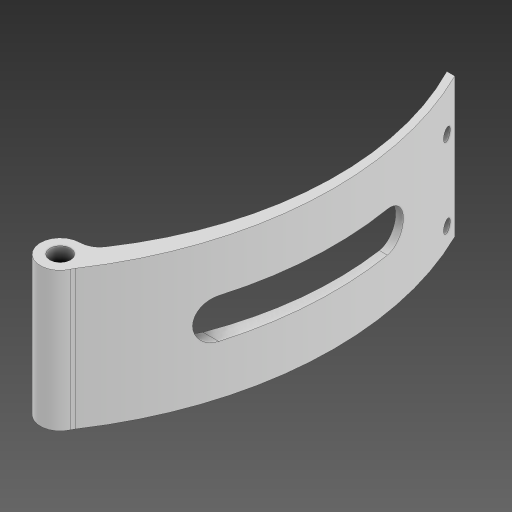
# Autodesk Inventor part: protect_2
Saved by Autodesk Inventor 2023 (Build 270158000, 158)
## iProperties
Created: 2025-06-27
Part Number: protect_2
Material: Типовые
Document SubType Name: Modeling
Designer: daa
Density: 1 g/cm^3
Appearance: По умолчанию
Author: daa
Autodesk Inventor part; units mm, degrees
ref_plane "YZ Plane" through (0, 0, 0) normal (1, 0, 0) x (0, 1, 0)
ref_plane "XZ Plane" through (0, 0, 0) normal (0, 1, 0) x (-1, 0, 0)
ref_plane "XY Plane" through (0, 0, 0) normal (0, 0, 1) x (1, 0, 0)
sketch "Эскиз1" plane through (0, 0, 0) normal (0, 1, 0) x (-1, 0, 0)
  circle A0 centre (-56.0718, 132.2835) radius 2.6
  line L0 (-64.9084, 43.85) -> (-66.9084, 43.85)
  circle A1 centre (-56.0718, 132.2835) radius 5.0026
  arc A2 (-60.8228, 133.85) -> (-66.9084, 43.85) centre (13.8399, 83.5958) ccw
  arc A3 (-58.2432, 127.7768) -> (-64.9084, 43.85) centre (6.2398, 80.4278) ccw
  line L1 (-60.8228, 133.85) -> (-51.3208, 133.85)
  point P0 (-68.2724, 116.2724)
  dimension "d27" = 5.2
  dimension "d28" = 2
  dimension "d29" = 90
  dimension "d30" = 80
  dimension "d35" = 90
  dimension "d47" = 10.0052
  dimension "d48" = 1.5665
  constraints: 7 point on circle, 4 centre point, 4 end point, 2 coincident, 2 horizontal
  measures "d27" diameter of A0
  measures "d28" distance of L0.start L0.end
  measures "d29" radius of A2
  measures "d30" radius of A3
  measures "d35" vertical distance of L0.end L1.start
  measures "d47" diameter of A1
  measures "d48" distance from line of L1 A0.centre
extrude "Выдавливание1" add sketch "Эскиз1" along normal blind 35 contours A0 L1 A1 | A0 L1 A1 | A1 A3 L0 A2
sketch "Эскиз2" plane through (0, 0, 0) normal (1, 0, 0) x (0, 1, 0)
  circle A0 centre (25, 47.55) radius 1.5
  circle A1 centre (5, 47.55) radius 1.5
  line L0 (0, 43.85) -> (35, 43.85) projected
  line L1 (35, 127.7768) -> (35, 43.85) projected
  line L2 (17.5, 68.85) -> (17.5, 108.85) construction
  line L3 (22.5, 68.85) -> (22.5, 108.85)
  line L4 (12.5, 108.85) -> (12.5, 68.85)
  arc A2 (12.5, 68.85) -> (22.5, 68.85) centre (17.5, 68.85) ccw
  arc A3 (22.5, 108.85) -> (12.5, 108.85) centre (17.5, 108.85) ccw
  point P0 (0, 0)
  point P1 (17.5, 88.85)
  point P2 (17.5, 63.85)
  dimension "d36" = 3
  dimension "d37" = 3
  dimension "d38" = 3.7
  dimension "d39" = 3.7
  dimension "d40" = 10
  dimension "d41" = 20
  dimension "d44" = 40
  dimension "d45" = 10
  dimension "d46" = 20
  constraints: 8 end point, 5 point on circle, 4 centre point, 4 tangent, 1 midpoint, 1 parallel, 1 vertical
  measures "d36" diameter of A0
  measures "d37" diameter of A1
  measures "d38" distance from line of L0 A1.centre
  measures "d39" distance from line of L0 A0.centre
  measures "d40" distance from line of L1 A0.centre
  measures "d41" distance of A0.centre A1.centre
  measures "d44" distance of L2.start L2.end
  measures "d45" diameter of A3
  measures "d46" distance from line of point (17.5, 63.85) L0
extrude "Выдавливание2" cut sketch "Эскиз2" along normal blind 94.5
fillet "Сопряжение3" radius 5 1 edges at (58.2432, 17.5, 127.7768)
fillet "Сопряжение4" radius 5 1 edges at (60.8228, 17.5, 133.85)
